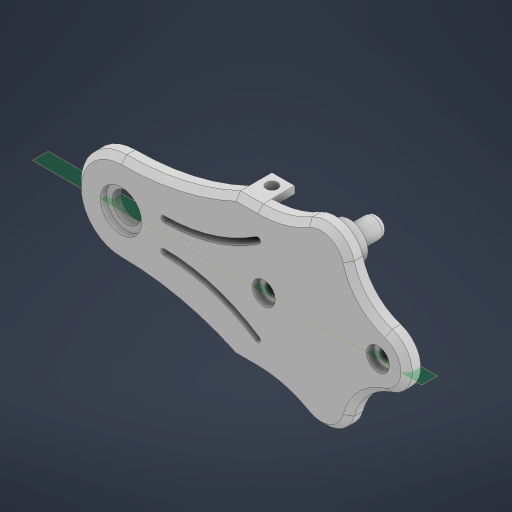
# Autodesk Inventor part: Bearing_Arm_2
Saved by Autodesk Inventor 2024.2 (Build 282272000, 272)
## iProperties
Created: 2024-04-12
Part Number: Bearing_Arm_2
Material: Generic
Document SubType Name: Modeling
Designer: CJ110
Density: 1 g/cm^3
Appearance: Default
Author: CJ110
## iProperties of the stored document Bearing_Arm_3DPrint.ipt
Created: 2024-04-12
Part Number: Bearing_Arm_3DPrint
Material: Generic
Document SubType Name: Modeling
Designer: jerem
Density: 1 g/cm^3
Appearance: Default
Author: jerem
Autodesk Inventor part; units mm, degrees
ref_plane "YZ Plane" through (0, 0, 0) normal (1, 0, 0) x (0, 1, 0)
ref_plane "XZ Plane" through (0, 0, 0) normal (0, 1, 0) x (-1, 0, 0)
ref_plane "XY Plane" through (0, 0, 0) normal (0, 0, 1) x (1, 0, 0)
sketch "Sketch1" plane through (0, 0, 0) normal (0, 0, 1) x (1, 0, 0)
  circle A0 centre (0, 0) radius 5.08
  arc A1 (0, 16) -> (0, -16) centre (0, 0) ccw
  line L0 (0, 16) -> (99.4033, 16)
  line L1 (99.4033, 16) -> (99.4033, -16)
  line L2 (99.4033, -16) -> (0, -16)
  line L3 (0, -16) -> (0, 16) construction
  line L4 (39.8634, 25) -> (99.4033, 25)
  line L5 (99.4033, 25) -> (99.4033, -25)
  line L6 (99.4033, -25) -> (39.8634, -25)
  line L7 (39.8634, -25) -> (39.8634, 25)
  arc A2 (39.8634, -25) -> (0, -16) centre (0, -108.7828) ccw
  arc A3 (0, 16) -> (39.8634, 25) centre (0, 108.7828) ccw
  circle A4 centre (50.0625, 0) radius 2
  circle A5 centre (90.0625, 0) radius 2
  line L8 (-16, 0) -> (99.4033, 0) construction
  point P0 (39.8634, 0)
  dimension "d1" = 10.16
  dimension "d3" = 50
  dimension "d4" = 59.5399
  dimension "d12" = 4
  dimension "d13" = 40
  dimension "d14" = 50.0625
  dimension "d15" = 9.3408
  dimension "d44" = 16
  constraints: 18 end point, 7 point on circle, 6 centre point, 4 parallel, 3 coincident, 3 horizontal, 3 midpoint, 3 tangent, 2 perpendicular, 2 point on line, 1 collinear, 1 equal radius, 1 horizontal alignment
  measures "d1" diameter of A0
  measures "d3" distance between parallel lines of L6 L4
  measures "d4" distance between parallel lines of L5 L7
  measures "d12" diameter of A5
  measures "d13" distance of A4.centre A5.centre
  measures "d14" distance of A0.centre A4.centre
  measures "d15" distance from line of L1 A5.centre
  measures "d44" radius of A1
extrude "Extrusion1" add sketch "Sketch1" along normal blind 5
ref_plane "Work Plane1" through (39.8634, 0, 0) normal (0, -1, 0) x (1, 0, 0)
sketch "Sketch4" plane through (0, 0, 5) normal (0, 0, 1) x (1, 0, 0)
  arc A0 (15, 6) -> (47.3064, 15.8305) centre (15, 64.0002) ccw
  arc A1 (15, 4) -> (48.4204, 14.1695) centre (15, 64.0002) ccw
  circle A2 centre (47.8634, 15) radius 1
  circle A3 centre (15, 5) radius 1
  arc A4 (0, 16) -> (39.8634, 25) centre (0, 108.7828) ccw projected
  line L0 (99.4033, 25) -> (39.8634, 25) projected
  line L1 (122.484, 0) -> (-39.0807, 0) projected
  line L2 (15, 4) -> (47.8634, 4) construction
  point P0 (0, 0)
  dimension "d16" = 2
  dimension "d17" = 10
  dimension "d18" = 8
  dimension "d19" = 15
  dimension "d20" = 5
  constraints: 8 point on circle, 5 tangent, 4 centre point, 2 end point, 1 concentric, 1 equal radius, 1 horizontal, 1 vertical alignment
  measures "d16" diameter of A2
  measures "d17" distance from line of L0 A2.centre
  measures "d18" horizontal distance of L0.end A2.centre
  measures "d19" horizontal distance of point (0, 0) A3.centre
  measures "d20" distance from line of L1 A3.centre
extrude "Extrusion3" cut sketch "Sketch4" against normal through all
mirror "Mirror1" about plane through (39.8634, 0, 0) normal (0, -1, 0) of "Extrusion3"
sketch "Sketch5" plane through (0, 0, 0) normal (0, 0, -1) x (-1, 0, 0)
  arc A0 (-15, -4) -> (-48.4204, -14.1695) centre (-15, -64.0002) ccw projected
  arc A1 (-15, -6) -> (-15, -4) centre (-15, -5) ccw projected
  arc A2 (-15, -6) -> (-47.3064, -15.8305) centre (-15, -64.0002) ccw projected
  arc A3 (-48.4204, -14.1695) -> (-47.3064, -15.8305) centre (-47.8634, -15) ccw projected
  arc A4 (-47.3064, 15.8305) -> (-15, 6) centre (-15, 64.0002) ccw projected
  arc A5 (-15, 4) -> (-15, 6) centre (-15, 5) ccw projected
  arc A6 (-48.4204, 14.1695) -> (-15, 4) centre (-15, 64.0002) ccw projected
  arc A7 (-47.3064, 15.8305) -> (-48.4204, 14.1695) centre (-47.8634, 15) ccw projected
  arc A8 (0, -16) -> (0, 16) centre (0, 0) ccw projected
  arc A9 (-39.8634, 25) -> (0, 16) centre (0, 108.7828) ccw projected
  line L0 (-99.4033, 25) -> (-39.8634, 25) projected
  line L1 (-99.4033, -25) -> (-99.4033, 25) projected
  line L2 (-39.8634, -25) -> (-99.4033, -25) projected
  arc A10 (0, -16) -> (-39.8634, -25) centre (0, -108.7828) ccw projected
  circle A11 centre (-50.0625, 0) radius 2 projected
  circle A12 centre (-90.0625, 0) radius 2 projected
  circle A13 centre (0, 0) radius 5.08 projected
  line L3 (-39.8634, 25) -> (-47.8634, 25)
  line L4 (-47.8634, 25) -> (-47.8634, 22.5)
  line L5 (-47.8634, 22.5) -> (-39.8634, 22.5)
  line L6 (-39.8634, 22.5) -> (-39.8634, 25)
  dimension "d23" = 8
  dimension "d24" = 2.5
  constraints: 8 end point, 2 parallel, 1 horizontal, 1 perpendicular
  measures "d23" distance of L4.end L5.end
  measures "d24" distance of L3.end L4.end
extrude "Extrusion4" add sketch "Sketch5" along normal blind 8 contours L6 L5 L4 L0
sketch "Sketch6" plane through (39.8634, 25, 5) normal (0, 1, 0) x (1, 0, 0)
  line L0 (59.5399, 5) -> (8, 5) projected
  line L1 (8, 5) -> (8, 13) projected
  line L2 (0, 13) -> (8, 13) projected
  line L3 (0, 5) -> (0, 13) projected
  line L4 (0, 5) -> (0, 0) projected
  line L5 (59.5399, 0) -> (0, 0) projected
  line L6 (59.5399, 5) -> (59.5399, 0) projected
  circle A0 centre (4, 9) radius 2
  line L7 (4, 13) -> (4, 9) construction
  point P0 (-39.8634, 5)
  dimension "d27" = 4
  dimension "d28" = 4
  constraints: 2 end point, 1 centre point, 1 midpoint, 1 vertical
  measures "d27" distance from line of L2 L7.end
  measures "d28" diameter of A0
extrude "Extrusion5" cut sketch "Sketch6" against normal up to next contours A0
mirror "Mirror2" about plane through (39.8634, 0, 0) normal (0, -1, 0) of "Extrusion4", "Extrusion5"
sketch "Sketch7" plane through (0, 0, 0) normal (0, 0, -1) x (-1, 0, 0)
  circle A0 centre (0, 0) radius 5.08 projected
  circle A1 centre (-90.0625, 0) radius 2 projected
  circle A2 centre (-50.0625, 0) radius 2 projected
  arc A3 (-47.3064, 15.8305) -> (-15, 6) centre (-15, 64.0002) ccw projected
  arc A4 (-15, 4) -> (-15, 6) centre (-15, 5) ccw projected
  arc A5 (-48.4204, 14.1695) -> (-15, 4) centre (-15, 64.0002) ccw projected
  arc A6 (-47.3064, 15.8305) -> (-48.4204, 14.1695) centre (-47.8634, 15) ccw projected
  arc A7 (-15, -4) -> (-48.4204, -14.1695) centre (-15, -64.0002) ccw projected
  arc A8 (-15, -6) -> (-15, -4) centre (-15, -5) ccw projected
  arc A9 (-15, -6) -> (-47.3064, -15.8305) centre (-15, -64.0002) ccw projected
  arc A10 (-48.4204, -14.1695) -> (-47.3064, -15.8305) centre (-47.8634, -15) ccw projected
  line L0 (-47.8634, -25) -> (-47.8634, -22.5) projected
  line L1 (-47.8634, -22.5) -> (-39.8634, -22.5) projected
  line L2 (-39.8634, -22.5) -> (-39.8634, -25) projected
  arc A11 (0, -16) -> (-39.8634, -25) centre (0, -108.7828) ccw projected
  arc A12 (0, -16) -> (0, 16) centre (0, 0) ccw projected
  arc A13 (-39.8634, 25) -> (0, 16) centre (0, 108.7828) ccw projected
  line L3 (-39.8634, 25) -> (-39.8634, 22.5) projected
  line L4 (-39.8634, 22.5) -> (-47.8634, 22.5) projected
  line L5 (-47.8634, 22.5) -> (-47.8634, 25) projected
  line L6 (-99.4033, 25) -> (-47.8634, 25) projected
  line L7 (-99.4033, -25) -> (-99.4033, 25) projected
  line L8 (-47.8634, -25) -> (-99.4033, -25) projected
  circle A14 centre (-70.0625, 21) radius 10
  arc A15 (-65.0249, 29.6384) -> (-47.8634, 25) centre (-47.8634, 59.0667) ccw
  line L9 (-99.4033, 25) -> (-47.8634, 25) projected
  line L10 (39.0807, 0) -> (-122.484, 0) projected
  line L11 (-70.0625, -25) -> (-70.0625, 21) construction
  line L12 (-90.0625, 0) -> (-50.0625, 0) construction
  line L13 (0, 16) -> (-99.4033, 16) construction
  arc A16 (-99.4033, 16) -> (-78.1686, 26.8559) centre (-99.4033, 42.1961) ccw
  point P0 (-92.2616, 25)
  point P1 (-75.1001, 29.6384)
  point P2 (-70.0625, 0)
  point P3 (-60.8973, 25)
  point P4 (-79.2277, 25)
  point P5 (-79.6415, 25)
  dimension "d31" = 20
  dimension "d32" = 21
  constraints: 7 point on circle, 6 end point, 5 tangent, 4 point on line, 3 centre point, 2 perpendicular, 1 coincident, 1 collinear, 1 midpoint, 1 vertical
  measures "d31" diameter of A14
  measures "d32" distance from line of L10 A14.centre
extrude "Extrusion6" add sketch "Sketch7" against normal up to surface (5 mm away) contours L6 A14 A15 | L6 A14 | A16 A14 L6 picked at (-67.4658, 26.7505)
sketch "Sketch8" plane through (0, 0, 0) normal (0, 0, -1) x (-1, 0, 0)
  circle A0 centre (0, 0) radius 5.08 projected
  circle A1 centre (-90.0625, 0) radius 2 projected
  circle A2 centre (-50.0625, 0) radius 2 projected
  arc A3 (-47.3064, 15.8305) -> (-15, 6) centre (-15, 64.0002) ccw projected
  arc A4 (-15, 4) -> (-15, 6) centre (-15, 5) ccw projected
  arc A5 (-48.4204, 14.1695) -> (-15, 4) centre (-15, 64.0002) ccw projected
  arc A6 (-47.3064, 15.8305) -> (-48.4204, 14.1695) centre (-47.8634, 15) ccw projected
  arc A7 (-15, -4) -> (-48.4204, -14.1695) centre (-15, -64.0002) ccw projected
  arc A8 (-15, -6) -> (-15, -4) centre (-15, -5) ccw projected
  arc A9 (-15, -6) -> (-47.3064, -15.8305) centre (-15, -64.0002) ccw projected
  arc A10 (-48.4204, -14.1695) -> (-47.3064, -15.8305) centre (-47.8634, -15) ccw projected
  line L0 (-47.8634, -25) -> (-47.8634, -22.5) projected
  line L1 (-47.8634, -22.5) -> (-39.8634, -22.5) projected
  line L2 (-39.8634, -22.5) -> (-39.8634, -25) projected
  arc A11 (0, -16) -> (-39.8634, -25) centre (0, -108.7828) ccw projected
  arc A12 (0, -16) -> (0, 16) centre (0, 0) ccw projected
  arc A13 (-39.8634, 25) -> (0, 16) centre (0, 108.7828) ccw projected
  line L3 (-39.8634, 25) -> (-39.8634, 22.5) projected
  line L4 (-39.8634, 22.5) -> (-47.8634, 22.5) projected
  line L5 (-47.8634, 22.5) -> (-47.8634, 25) projected
  arc A14 (-65.0249, 29.6384) -> (-47.8634, 25) centre (-47.8634, 59.0667) ccw projected
  arc A15 (-65.0249, 29.6384) -> (-78.1686, 26.8559) centre (-70.0625, 21) ccw projected
  line L6 (-99.4033, 25) -> (-79.6415, 25) projected
  line L7 (-99.4033, -25) -> (-99.4033, 25) projected
  line L8 (-47.8634, -25) -> (-99.4033, -25) projected
  circle A16 centre (-70.0625, 21) radius 6.5
  arc A17 (-79.6415, 25) -> (-78.1686, 26.8559) centre (-99.4033, 42.1961) ccw projected
  dimension "d35" = 13
  constraints: 1 centre point, 1 coincident
  measures "d35" diameter of A16
extrude "Extrusion7" add sketch "Sketch8" along normal blind 5 contours A16
sketch "Sketch9" plane through (70.0625, 21, -5) normal (0, 0, -1) x (-1, 0, 0)
  circle A0 centre (0, 0) radius 3.5
  circle A1 centre (0, 0) radius 6.5 projected
  point P0 (70.0625, -21)
  dimension "d38" = 7
  constraints: 1 centre point, 1 coincident
  measures "d38" diameter of A0
extrude "Extrusion8" add sketch "Sketch9" along normal blind 10 contours A0
fillet "Fillet1" radius 2 1 edges at (73.5625, 21, -15)
extrude "Extrusion9" cut sketch "Sketch7" against normal through all contours L7 L6 A16
mirror "Mirror3" about plane through (39.8634, 0, 0) normal (0, -1, 0) of "Extrusion6", "Extrusion7", "Extrusion8", "Fillet1", "Extrusion9"
sketch "Sketch10" plane through (0, 0, 5) normal (0, 0, 1) x (1, 0, 0)
  arc A0 (48.4204, -14.1695) -> (15, -4) centre (15, -64.0002) ccw projected
  arc A1 (47.3064, -15.8305) -> (48.4204, -14.1695) centre (47.8634, -15) ccw projected
  arc A2 (47.3064, -15.8305) -> (15, -6) centre (15, -64.0002) ccw projected
  arc A3 (15, -4) -> (15, -6) centre (15, -5) ccw projected
  arc A4 (15, 6) -> (47.3064, 15.8305) centre (15, 64.0002) ccw projected
  arc A5 (48.4204, 14.1695) -> (47.3064, 15.8305) centre (47.8634, 15) ccw projected
  arc A6 (15, 4) -> (48.4204, 14.1695) centre (15, 64.0002) ccw projected
  arc A7 (15, 6) -> (15, 4) centre (15, 5) ccw projected
  arc A8 (99.4033, -16) -> (78.1686, -26.8559) centre (99.4033, -42.1961) ccw projected
  line L0 (99.4033, -16) -> (99.4033, 16) projected
  arc A9 (78.1686, 26.8559) -> (99.4033, 16) centre (99.4033, 42.1961) ccw projected
  line L1 (47.8634, 25) -> (39.8634, 25) projected
  arc A10 (78.1686, 26.8559) -> (65.0249, 29.6384) centre (70.0625, 21) ccw projected
  arc A11 (47.8634, 25) -> (65.0249, 29.6384) centre (47.8634, 59.0667) ccw projected
  arc A12 (0, 16) -> (39.8634, 25) centre (0, 108.7828) ccw projected
  arc A13 (0, 16) -> (0, -16) centre (0, 0) ccw projected
  arc A14 (39.8634, -25) -> (0, -16) centre (0, -108.7828) ccw projected
  line L2 (39.8634, -25) -> (47.8634, -25) projected
  arc A15 (65.0249, -29.6384) -> (47.8634, -25) centre (47.8634, -59.0667) ccw projected
  arc A16 (65.0249, -29.6384) -> (78.1686, -26.8559) centre (70.0625, -21) ccw projected
  circle A17 centre (50.0625, 0) radius 2 projected
  circle A18 centre (90.0625, 0) radius 2 projected
  circle A19 centre (0, 0) radius 5.08 projected
  circle A20 centre (50.0625, 0) radius 4
  circle A21 centre (90.0625, 0) radius 4
  dimension "d45" = 8
  constraints: 2 centre point, 2 coincident, 1 equal radius
  measures "d45" diameter of A21
extrude "Extrusion10" cut sketch "Sketch10" against normal blind 2.5 contours A20 | A21
sketch "Sketch11" plane through (0, 0, 5) normal (0, 0, 1) x (1, 0, 0)
  circle A0 centre (0, 0) radius 7.235
  dimension "d48" = 14.47
  constraints: 1 centre point, 1 coincident
  measures "d48" diameter of A0
extrude "Extrusion11" cut sketch "Sketch11" against normal blind 2
sketch "Sketch12" plane through (0, 0, 0) normal (0, 0, -1) x (-1, 0, 0)
  circle A0 centre (-70.0625, 21) radius 1.5 projected
  circle A1 centre (-70.0625, 21) radius 10
  circle A2 centre (-90.0625, 0) radius 2 projected
  circle A3 centre (-90.0625, 0) radius 10
  circle A4 centre (-70.0625, -21) radius 1.5 projected
  circle A5 centre (-70.0625, -21) radius 10
  circle A6 centre (-90.0625, 0) radius 2
  arc A7 (-79.7352, -23.5375) -> (-93.0685, -9.5375) centre (-99.0806, -28.6125) ccw
  arc A8 (-93.0685, 9.5375) -> (-79.7352, 23.5375) centre (-99.0806, 28.6125) ccw
  arc A9 (-78.1686, -26.8559) -> (-99.4033, -16) centre (-99.4033, -42.1961) ccw projected
  arc A10 (-78.1686, -26.8559) -> (-65.0249, -29.6384) centre (-70.0625, -21) ccw projected
  arc A11 (-47.8634, -25) -> (-65.0249, -29.6384) centre (-47.8634, -59.0667) ccw projected
  line L0 (-47.8634, -25) -> (-47.8634, -22.5) projected
  line L1 (-47.8634, -22.5) -> (-39.8634, -22.5) projected
  line L2 (-39.8634, -22.5) -> (-39.8634, -25) projected
  arc A12 (0, -16) -> (-39.8634, -25) centre (0, -108.7828) ccw projected
  arc A13 (0, -16) -> (0, 16) centre (0, 0) ccw projected
  arc A14 (-39.8634, 25) -> (0, 16) centre (0, 108.7828) ccw projected
  line L3 (-39.8634, 25) -> (-39.8634, 22.5) projected
  line L4 (-39.8634, 22.5) -> (-47.8634, 22.5) projected
  line L5 (-47.8634, 22.5) -> (-47.8634, 25) projected
  arc A15 (-65.0249, 29.6384) -> (-47.8634, 25) centre (-47.8634, 59.0667) ccw projected
  arc A16 (-65.0249, 29.6384) -> (-78.1686, 26.8559) centre (-70.0625, 21) ccw projected
  arc A17 (-99.4033, 16) -> (-78.1686, 26.8559) centre (-99.4033, 42.1961) ccw projected
  line L6 (-99.4033, -16) -> (-99.4033, 16) projected
  circle A18 centre (-70.0625, -21) radius 6.5 projected
  circle A19 centre (-70.0625, 21) radius 6.5 projected
  circle A20 centre (0, 0) radius 5.08 projected
  circle A21 centre (-90.0625, 0) radius 2 projected
  circle A22 centre (-50.0625, 0) radius 2 projected
  arc A23 (-47.3064, 15.8305) -> (-15, 6) centre (-15, 64.0002) ccw projected
  arc A24 (-15, 4) -> (-15, 6) centre (-15, 5) ccw projected
  arc A25 (-48.4204, 14.1695) -> (-15, 4) centre (-15, 64.0002) ccw projected
  arc A26 (-47.3064, 15.8305) -> (-48.4204, 14.1695) centre (-47.8634, 15) ccw projected
  arc A27 (-15, -4) -> (-48.4204, -14.1695) centre (-15, -64.0002) ccw projected
  arc A28 (-15, -6) -> (-15, -4) centre (-15, -5) ccw projected
  arc A29 (-15, -6) -> (-47.3064, -15.8305) centre (-15, -64.0002) ccw projected
  arc A30 (-48.4204, -14.1695) -> (-47.3064, -15.8305) centre (-47.8634, -15) ccw projected
  point P0 (-99.4033, -3.5706)
  point P1 (-99.4033, 3.5706)
  dimension "d54" = 20
  dimension "d56" = 20
  dimension "d55" = 20
  dimension "d57" = 4
  dimension "d58" = 20
  dimension "d59" = 20
  constraints: 6 point on circle, 4 centre point, 4 coincident, 2 tangent, 8 other
  measures "d55" diameter of A3
  measures "d57" diameter of A6
  measures "d58" radius of A8
  measures "d59" radius of A7
extrude "Extrusion12" cut sketch "Sketch12" against normal blind 10 contours A8 A3 L6 A17 A1 | A7 A5 A9 L6 A3
extrude "Extrusion13" add sketch "Sketch12" against normal up to surface (5 mm away) contours L6 A3 picked at (-99.5984, 0.4047)
chamfer "Chamfer1" distance 2 angle 45 5 edges at (20.4334, 18.278, 5) (-16, 0, 5) (20.4334, -18.278, 5) (43.8634, 25, 5) (43.8634, -25, 5)
equation "\"d59\" = d58"
body "Solid1"
